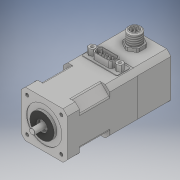
# Autodesk Inventor part: 1460675 EMMS-ST-42-SS-SE-G2
Saved by Autodesk Inventor 2019 (Build 230136000, 136)
## iProperties
Created: 2023-04-07
Part Number: 1460675 EMMS-ST-42-SS-SE-G2
Material: Generic
Catalog Web Link: www.cadenas.de
Description: EMMS-ST-SS-stepper motor
Vendor: FESTO
Document SubType Name: Modeling
Designer: psAdmin
Manufacturer: FESTO
Mass: 450 g
Surface Area: 209.206 cm^2
Volume: 162.575 cm^3
Density: 1 g/cm^3
Appearance: PSOLRGB-175-175-175
Category: PARTsolutions
Company: FESTO
Title: 1460675 EMMS-ST-42-SS-SE-G2
Author: Cadenas PARTsolutions
Comments: stepper motor
PSOL_IDENT_0: {$CADENAS_DATA/23d-libs/festo/parts/e/emms/emms_st_ss.prj},200 {VTYP=3D},{NB=1460675 EMMS-ST-42-SS-S
PSOL_IDENT_1: E-G2},{LINA=1460675 EMMS-ST-42-SS-SE-G2},{NN=EMMS-ST-SS},{DATE=13.09.2021 11:28:07},{GEOMDATE=11.09.
PSOL_IDENT_2: 2019 11:09:23},{VERSION=},{LINEID=1120},{WBVAR=},{WBNUMERIC=}  {NB=1460675 EMMS-ST-42-SS-SE-G2},{LIN
PSOL_IDENT_3: A=1460675 EMMS-ST-42-SS-SE-G2},{KT=DUMMY},{TNR=1460675},{TYP=EMMS-ST-42-SS-SE-G2},{A=94.000},{B=M12}
PSOL_IDENT_4: ,{C=13.000},{D=6.500},{MES=2.000},{BRE=1.000},{VER=2.000},{VERS=2},{DP=1},{L=64.0},{L1=11.0},{L2=30.
PSOL_IDENT_5: 0},{L3=2.0},{L4=40.0},{L5=17},{L6=6.5},{L7=24.0},{L8=0.00},{H=38},{H1=13},{H2=0},{D1=22.0},{D2=5.00}
PSOL_IDENT_6: ,{D3=31.00},{D4=42.0},{D5=0.0},{M=M3},{MA=3.000},{M1=M12},{M1A=12.000},{CNSMASSEXACT=0.4500}
NB: 1460675 EMMS-ST-42-SS-SE-G2
NN: EMMS-ST-SS
NT: stepper motor
NBSYN: $TNR. $TYP.
LINA: 1460675 EMMS-ST-42-SS-SE-G2
CATALOG: Festo
TNR: 1460675
TYP: EMMS-ST-42-SS-SE-G2
A: 94
B: M12
C: 13
D: 6.5
CNSMASSEXACT: 0.45
SUPPLIER: FESTO
ARTICLENO: 1460675 EMMS-ST-42-SS-SE-G2
BOMINFO: 1460675 EMMS-ST-42-SS-SE-G2
CREATOR: CADENAS GmbH
Autodesk Inventor part; units mm, degrees
sketch "Sketch_1" plane through (0, 0, 0) normal (0, 1, 0) x (-1, 0, 0)
  line L0 (0, 11) -> (0, -2)
  line L1 (0, -2) -> (-11, -2)
  line L2 (-11, -2) -> (-11, 2)
  line L3 (-11, 2) -> (-2.5, 2)
  line L4 (-2.5, 2) -> (-2.5, 10.8)
  line L5 (-2.5, 10.8) -> (-2.3, 11)
  line L6 (-2.3, 11) -> (0, 11)
  line L7 (0, 11) -> (0, -2)
  constraints: 16 end point
revolve "Revolution1" add sketch "Sketch_1" angle 360 about axis through (0, 0, 11) along (0, 0, 1)
sketch "Sketch_2" plane through (0, 0, 0) normal (0, 0, 1) x (1, 0, 0)
  line L0 (-21, 16.9706) -> (-21, -16.9706)
  arc A0 (-21, -16.9706) -> (-16.9706, -21) centre (0, 0) ccw
  line L1 (-16.9706, -21) -> (16.9706, -21)
  arc A1 (16.9706, -21) -> (21, -16.9706) centre (0, 0) ccw
  line L2 (21, -16.9706) -> (21, 16.9706)
  arc A2 (21, 16.9706) -> (16.9706, 21) centre (0, 0) ccw
  line L3 (16.9706, 21) -> (-16.9706, 21)
  arc A3 (-16.9706, 21) -> (-21, 16.9706) centre (0, 0) ccw
  constraints: 8 end point, 8 point on circle, 4 centre point
extrude "Extrusion1" add sketch "Sketch_2" against normal blind 64
sketch "Sketch_12" plane through (0, 0, 0) normal (0, 1, 0) x (-1, 0, 0)
  line L0 (0, 50) -> (0, -50)
  line L1 (-11, -0.5) -> (-11, 0)
  line L2 (-11, 0) -> (-16, 0)
  line L3 (-16, 0) -> (-16, -0.5)
  line L4 (-16, -0.5) -> (-11, -0.5)
  constraints: 10 end point
revolve "Revolution2" cut sketch "Sketch_12" angle 360 about axis through (0, 0, 50) along (0, 0, 1)
sketch "Sketch_3" plane through (0, 0, -38.2) normal (0, 0, 1) x (1, 0, 0)
  line L0 (-25.2, 25.2) -> (-25.2, -25.2)
  line L1 (-25.2, -25.2) -> (25.2, -25.2)
  line L2 (25.2, -25.2) -> (25.2, 25.2)
  line L3 (25.2, 25.2) -> (-25.2, 25.2)
  line L4 (-21, 12.1127) -> (-21, -12.1127)
  arc A0 (-21, -12.1127) -> (-20.4142, -13.5269) centre (-19, -12.1127) ccw
  line L5 (-20.4142, -13.5269) -> (-13.5269, -20.4142)
  arc A1 (-13.5269, -20.4142) -> (-12.1127, -21) centre (-12.1127, -19) ccw
  line L6 (-12.1127, -21) -> (12.1127, -21)
  arc A2 (12.1127, -21) -> (13.5269, -20.4142) centre (12.1127, -19) ccw
  line L7 (13.5269, -20.4142) -> (20.4142, -13.5269)
  arc A3 (20.4142, -13.5269) -> (21, -12.1127) centre (19, -12.1127) ccw
  line L8 (21, -12.1127) -> (21, 12.1127)
  arc A4 (21, 12.1127) -> (20.4142, 13.5269) centre (19, 12.1127) ccw
  line L9 (20.4142, 13.5269) -> (13.5269, 20.4142)
  arc A5 (13.5269, 20.4142) -> (12.1127, 21) centre (12.1127, 19) ccw
  line L10 (12.1127, 21) -> (-12.1127, 21)
  arc A6 (-12.1127, 21) -> (-13.5269, 20.4142) centre (-12.1127, 19) ccw
  line L11 (-13.5269, 20.4142) -> (-20.4142, 13.5269)
  arc A7 (-20.4142, 13.5269) -> (-21, 12.1127) centre (-19, 12.1127) ccw
  constraints: 24 end point, 16 point on circle, 8 centre point
extrude "Extrusion2" cut sketch "Sketch_3" along normal blind 27.2
sketch "Sketch_6" plane through (0, 0, -64) normal (0, 0, 1) x (1, 0, 0)
  line L0 (-20.9, 17.0936) -> (-20.9, -17.0936)
  arc A0 (-20.9, -17.0936) -> (-16.8461, -21.1) centre (0, 0) ccw
  line L1 (-16.8461, -21.1) -> (16.8461, -21.1)
  arc A1 (16.8461, -21.1) -> (20.9, -17.0936) centre (0, 0) ccw
  line L2 (20.9, -17.0936) -> (20.9, 17.0936)
  arc A2 (20.9, 17.0936) -> (16.8461, 21.1) centre (0, 0) ccw
  line L3 (16.8461, 21.1) -> (-16.8461, 21.1)
  arc A3 (-16.8461, 21.1) -> (-20.9, 17.0936) centre (0, 0) ccw
  constraints: 8 end point, 8 point on circle, 4 centre point
extrude "Extrusion3" add sketch "Sketch_6" against normal blind 30
sketch "Sketch6" plane through (0, 0, 0) normal (0, 0, 1) x (1, 0, 0)
  point P0 (15.5, -15.5)
hole "Hole1" at (15.5, -15.5, 0) direction (0, 0, -1) diameter 2.459 depth 4.5 tip angle 120 countersink diameter 3 countersink angle 90 thread size "M3x0.5" class "6H" standard "ISO Metric profile"
sketch "Sketch7" plane through (0, 0, 0) normal (0, 0, 1) x (1, 0, 0)
  point P0 (-15.5, -15.5)
hole "Hole2" at (-15.5, -15.5, 0) direction (0, 0, -1) diameter 2.459 depth 4.5 tip angle 120 countersink diameter 3 countersink angle 90 thread size "M3x0.5" class "6H" standard "ISO Metric profile"
sketch "Sketch8" plane through (0, 0, 0) normal (0, 0, 1) x (1, 0, 0)
  point P0 (15.5, 15.5)
hole "Hole3" at (15.5, 15.5, 0) direction (0, 0, -1) diameter 2.459 depth 4.5 tip angle 120 countersink diameter 3 countersink angle 90 thread size "M3x0.5" class "6H" standard "ISO Metric profile"
sketch "Sketch9" plane through (0, 0, 0) normal (0, 0, 1) x (1, 0, 0)
  point P0 (-15.5, 15.5)
hole "Hole4" at (-15.5, 15.5, 0) direction (0, 0, -1) diameter 2.459 depth 4.5 tip angle 120 countersink diameter 3 countersink angle 90 thread size "M3x0.5" class "6H" standard "ISO Metric profile"
sketch "Sketch_13" plane through (0, 21, 0) normal (0, 1, 0) x (1, 0, 0)
  arc A0 (-7.4384, 60) -> (-9.3787, 57.5149) centre (-7.4384, 58) ccw
  line L0 (-9.3787, 57.5149) -> (-8.3787, 53.5149)
  arc A1 (-8.3787, 53.5149) -> (-6.4384, 52) centre (-6.4384, 54) ccw
  line L1 (-6.4384, 52) -> (6.4384, 52)
  arc A2 (6.4384, 52) -> (8.3787, 53.5149) centre (6.4384, 54) ccw
  line L2 (8.3787, 53.5149) -> (9.3787, 57.5149)
  arc A3 (9.3787, 57.5149) -> (7.4384, 60) centre (7.4384, 58) ccw
  line L3 (7.4384, 60) -> (-7.4384, 60)
  constraints: 8 end point, 8 point on circle, 4 centre point
extrude "Extrusion4" add sketch "Sketch_13" along normal blind 6.5
sketch "Sketch_14" plane through (0, 21, 0) normal (0, 1, 0) x (1, 0, 0)
  line L0 (-16, 61) -> (-16, 51)
  arc A0 (-16, 51) -> (-15, 50) centre (-15, 51) ccw
  line L1 (-15, 50) -> (15, 50)
  arc A1 (15, 50) -> (16, 51) centre (15, 51) ccw
  line L2 (16, 51) -> (16, 61)
  arc A2 (16, 61) -> (15, 62) centre (15, 61) ccw
  line L3 (15, 62) -> (-15, 62)
  arc A3 (-15, 62) -> (-16, 61) centre (-15, 61) ccw
  constraints: 8 end point, 8 point on circle, 4 centre point
extrude "Extrusion5" add sketch "Sketch_14" along normal blind 0.6
sketch "Sketch_21" plane through (0, 21.6, 0) normal (0, 1, 0) x (1, 0, 0)
  arc A0 (-6.662, 59.5) -> (-8.5455, 56.8273) centre (-6.662, 57.5) ccw
  line L0 (-8.5455, 56.8273) -> (-7.474, 53.8273)
  arc A1 (-7.474, 53.8273) -> (-5.5906, 52.5) centre (-5.5906, 54.5) ccw
  line L1 (-5.5906, 52.5) -> (5.5906, 52.5)
  arc A2 (5.5906, 52.5) -> (7.474, 53.8273) centre (5.5906, 54.5) ccw
  line L2 (7.474, 53.8273) -> (8.5455, 56.8273)
  arc A3 (8.5455, 56.8273) -> (6.662, 59.5) centre (6.662, 57.5) ccw
  line L3 (6.662, 59.5) -> (-6.662, 59.5)
  circle A4 centre (5, 57) radius 0.5
  circle A5 centre (3.75, 54.5) radius 0.5
  circle A6 centre (2.5, 57) radius 0.5
  circle A7 centre (1.25, 54.5) radius 0.5
  circle A8 centre (0, 57) radius 0.5
  circle A9 centre (-1.25, 54.5) radius 0.5
  circle A10 centre (-2.5, 57) radius 0.5
  circle A11 centre (-3.75, 54.5) radius 0.5
  circle A12 centre (-5, 57) radius 0.5
  constraints: 13 centre point, 8 end point, 8 point on circle
extrude "Extrusion6" cut sketch "Sketch_21" along normal blind 5.9
sketch "Sketch_15" plane through (0, 21, 0) normal (0, 1, 0) x (1, 0, 0)
  line L0 (9.75, 54.4123) -> (12.5, 52.8246)
  line L1 (12.5, 52.8246) -> (15.25, 54.4123)
  line L2 (15.25, 54.4123) -> (15.25, 57.5877)
  line L3 (15.25, 57.5877) -> (12.5, 59.1754)
  line L4 (12.5, 59.1754) -> (9.75, 57.5877)
  line L5 (9.75, 57.5877) -> (9.75, 54.4123)
  circle A0 centre (12.5, 56) radius 1.25
  constraints: 12 end point, 1 centre point
extrude "Extrusion7" add sketch "Sketch_15" along normal blind 6
sketch "Sketch_16" plane through (0, 21, 0) normal (0, 1, 0) x (1, 0, 0)
  line L0 (-15.25, 54.4123) -> (-12.5, 52.8246)
  line L1 (-12.5, 52.8246) -> (-9.75, 54.4123)
  line L2 (-9.75, 54.4123) -> (-9.75, 57.5877)
  line L3 (-9.75, 57.5877) -> (-12.5, 59.1754)
  line L4 (-12.5, 59.1754) -> (-15.25, 57.5877)
  line L5 (-15.25, 57.5877) -> (-15.25, 54.4123)
  circle A0 centre (-12.5, 56) radius 1.25
  constraints: 12 end point, 1 centre point
extrude "Extrusion8" add sketch "Sketch_16" along normal blind 6
sketch "Sketch_17" plane through (0, 0, -94) normal (0, 0, 1) x (1, 0, 0)
  line L0 (-8.5, -19) -> (8.5, -19)
  line L1 (8.5, -19) -> (8.5, 19)
  line L2 (8.5, 19) -> (-8.5, 19)
  line L3 (-8.5, 19) -> (-8.5, -19)
  constraints: 8 end point
extrude "Extrusion9" cut sketch "Sketch_17" along normal blind 0.1
sketch "Sketch_19" plane through (0, 21, 0) normal (0, 1, 0) x (1, 0, 0)
  line L0 (-7, 84.8868) -> (-7, 79.1132)
  arc A0 (-7, 79.1132) -> (-6, 77.3812) centre (-5, 79.1132) ccw
  line L1 (-6, 77.3812) -> (-1, 74.4944)
  arc A1 (-1, 74.4944) -> (1, 74.4944) centre (0, 76.2265) ccw
  line L2 (1, 74.4944) -> (6, 77.3812)
  arc A2 (6, 77.3812) -> (7, 79.1132) centre (5, 79.1132) ccw
  line L3 (7, 79.1132) -> (7, 84.8868)
  arc A3 (7, 84.8868) -> (6, 86.6188) centre (5, 84.8868) ccw
  line L4 (6, 86.6188) -> (1, 89.5056)
  arc A4 (1, 89.5056) -> (-1, 89.5056) centre (0, 87.7735) ccw
  line L5 (-1, 89.5056) -> (-6, 86.6188)
  arc A5 (-6, 86.6188) -> (-7, 84.8868) centre (-5, 84.8868) ccw
  constraints: 12 end point, 12 point on circle, 6 centre point
extrude "Extrusion10" add sketch "Sketch_19" along normal blind 3
sketch "Sketch_20" plane through (0, 0, 0) normal (1, 0, 0) x (0, 1, 0)
  line L0 (21, -82) -> (34.1, -82)
  line L1 (34.1, -82) -> (34.1, -86.9265)
  line L2 (34.1, -86.9265) -> (33.0265, -88)
  line L3 (33.0265, -88) -> (21, -88)
  line L4 (21, -88) -> (21, -82)
  line L5 (21, -82) -> (34.1, -82)
  constraints: 12 end point
revolve "Revolution3" add sketch "Sketch_20" angle 360 about axis through (0, 21, -82) along (0, -1, 0)
thread "Thread1" size "M12x1.75" class "6g" standard "ISO Metric profile" length 8.9265
sketch "Sketch_22" plane through (0, 34.1, -82) normal (0, 1, 0) x (0, 0, -1)
  arc A0 (-3.9724, -0.4693) -> (-3.9724, 0.4693) centre (-3.8, 0) ccw
  arc A1 (-3.9724, -0.4693) -> (-3.9724, 0.4693) centre (0, 0) ccw
  circle A2 centre (2.7, 0) radius 0.5
  circle A3 centre (1.6834, 2.1109) radius 0.5
  circle A4 centre (1.6834, -2.1109) radius 0.5
  circle A5 centre (0, 0) radius 0.5
  circle A6 centre (-0.6008, 2.6323) radius 0.5
  circle A7 centre (-0.6008, -2.6323) radius 0.5
  circle A8 centre (-2.4326, 1.1715) radius 0.5
  circle A9 centre (-2.4326, -1.1715) radius 0.5
  constraints: 10 centre point, 4 point on circle
extrude "Extrusion11" cut sketch "Sketch_22" against normal blind 8
sketch "Sketch_23" plane through (0, 0, 0) normal (1, 0, 0) x (0, 1, 0)
  line L0 (0, -50) -> (0, 50)
  line L1 (5, 13) -> (2.5, 13)
  line L2 (2.5, 13) -> (2.5, -1)
  line L3 (2.5, -1) -> (5, -1)
  line L4 (5, -1) -> (5, 13)
  constraints: 10 end point
revolve "Revolution4" cut sketch "Sketch_23" angle 360 about axis through (0, 0, -50) along (0, 0, -1)
ref_plane "ANBAU_XY" through (0, 0, 0) normal (0, 0, -1) x (1, 0, 0)
ref_plane "ANBAU_YZ" through (0, 0, 0) normal (1, 0, 0) x (0, -1, 0)
ref_plane "ANBAU_ZX" through (0, 0, 0) normal (0, -1, 0) x (0, 0, -1)
ref_plane "EL_XY" through (0, 23.9, -82) normal (0, -1, 0) x (1, 0, 0)
ref_plane "EL_YZ" through (0, 23.9, -82) normal (1, 0, 0) x (0, 0, 1)
ref_plane "EL_ZX" through (0, 23.9, -82) normal (0, 0, 1) x (0, -1, 0)
ref_plane "ML_XY" through (0, 21.6, -56) normal (0, -1, 0) x (1, 0, 0)
ref_plane "ML_YZ" through (0, 21.6, -56) normal (1, 0, 0) x (0, 0, 1)
ref_plane "ML_ZX" through (0, 21.6, -56) normal (0, 0, 1) x (0, -1, 0)
body "Solid1"
